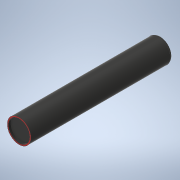
# Autodesk Inventor part: ueda_seal
Saved by Autodesk Inventor 2020.3 (Build 243373000, 373)
## iProperties
Created: 2020-10-19
Part Number: ueda_seal
Material: 一般
Document SubType Name: Modeling
Designer: Masato
Density: 1 g/cm^3
Appearance: 既定
Author: Masato
## iProperties of the stored document ueda_hanko_3D プリント.ipt
Created: 2020-10-19
Part Number: ueda_hanko_3D プリント
Material: 一般
Document SubType Name: Modeling
Designer: Masato
Density: 1 g/cm^3
Appearance: 既定
Author: Masato
Autodesk Inventor part; units mm, degrees
ref_plane "YZ Plane" through (0, 0, 0) normal (1, 0, 0) x (0, 1, 0)
ref_plane "XZ Plane" through (0, 0, 0) normal (0, 1, 0) x (-1, 0, 0)
sketch "スケッチ1" plane through (0, 0, 0) normal (0, 0, 1) x (1, 0, 0)
  circle A0 centre (0, 0) radius 5
  circle A1 centre (0, 0) radius 4.5
  dimension "d0" = 10
  dimension "d10" = 9
  constraints: 2 centre point, 2 coincident
  measures "d0" diameter of A0
  measures "d10" diameter of A1
ref_plane "作業平面1" through (0, 0, 0) normal (0, 0, -1) x (-1, 0, 0)
extrude "押し出し5" add sketch "スケッチ1" against normal blind 1
sketch "スケッチ3" plane through (0, 0, -1) normal (0, 0, -1) x (-1, 0, 0)
  circle A0 centre (0, 0) radius 5
  constraints: 1 centre point, 1 coincident
extrude "押し出し6" add sketch "スケッチ3" along normal blind 59
fillet "フィレット2" radius 1 1 edges at (5, 0, -60)
